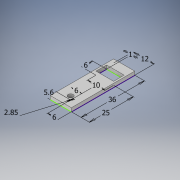
# Autodesk Inventor part: ir holder
Saved by Autodesk Inventor 2019.4 (Build 234330000, 330)
## iProperties
Created: 2021-06-18
Part Number: ir holder
Material: Generic
Document SubType Name: Modeling
Designer: marcu
Density: 1 g/cm^3
Appearance: Default
Author: marcu
Autodesk Inventor part; units mm, degrees
ref_plane "YZ Plane" through (0, 0, 0) normal (1, 0, 0) x (0, 1, 0)
ref_plane "XZ Plane" through (0, 0, 0) normal (0, 1, 0) x (-1, 0, 0)
ref_plane "XY Plane" through (0, 0, 0) normal (0, 0, 1) x (1, 0, 0)
sketch "Sketch1" plane through (0, 0, 0) normal (0, 1, 0) x (-1, 0, 0)
  line L0 (6, 21.6828) -> (-6, 21.6828)
  line L1 (-6, 21.6828) -> (-6, -14.3172)
  line L2 (-6, -14.3172) -> (6, -14.3172)
  line L3 (6, -14.3172) -> (6, 21.6828)
  line L4 (5, -3.3172) -> (-5, -3.3172)
  line L5 (-5, -3.3172) -> (-5, -9.3172)
  line L6 (-5, -9.3172) -> (5, -9.3172)
  line L7 (5, -9.3172) -> (5, -3.3172)
  circle A0 centre (0, 16.0828) radius 1.425
  point P0 (0, 0)
  dimension "d0" = 2.85
  dimension "d1" = 36
  dimension "d2" = 10
  dimension "d3" = 1
  dimension "d4" = 6
  dimension "d5" = 12
  dimension "d6" = 6
  dimension "d8" = 5.6
  dimension "d9" = 25
  dimension "d11" = 6
  constraints: 16 end point, 4 parallel, 2 horizontal, 2 perpendicular, 1 centre point
  measures "d0" diameter of A0
  measures "d1" distance of L0.end L1.end
  measures "d2" distance of L4.start L4.end
  measures "d3" distance between parallel lines of L7 L3
  measures "d4" distance from line of A0.centre L3
  measures "d5" distance of L1.end L2.end
  measures "d6" distance from line of L1 point (0, 0)
  measures "d8" distance from line of L0 A0.centre
  measures "d9" distance between parallel lines of L0 L4
  measures "d11" distance of L6.end L4.start
extrude "Extrusion1" add sketch "Sketch1" along normal blind 2
body "Solid1"
